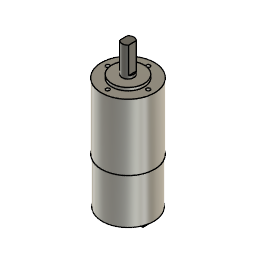
Motor 36GP-3530 (Autodesk Fusion 360 design; units mm, degrees)
Autodesk Fusion 360 part; units mm, degrees
sketch "Sketch1" plane through (0, 0, 0) normal (0, 0, 1) x (1, 0, 0)
  circle A0 centre (0, 0) radius 17.5
  circle A1 centre (0, 0) radius 18
  line L0 (0, 0) -> (11.5, 0) construction
  line L1 (0, 1) -> (0, -1) construction
  line L2 (12, 2) -> (11, 2)
  line L3 (11, 2) -> (11, -2)
  line L4 (11, -2) -> (12, -2)
  line L5 (12, -2) -> (12, 2)
  line L6 (12, 2) -> (11, -2) construction
  line L7 (11, 2) -> (12, -2) construction
  line L8 (-11, 2) -> (-11, -2)
  line L9 (-11, -2) -> (-12, -2)
  line L10 (-12, -2) -> (-12, 2)
  line L11 (-12, 2) -> (-11, 2)
  circle A2 centre (0, 0) radius 11
  circle A3 centre (0, 0) radius 4
  line L12 (-3, 2.6458) -> (-3, -2.6458)
  line L13 (3, -2.6458) -> (3, 2.6458)
  line L14 (3, 2.6458) -> (-3, -2.6458) construction
  line L15 (-3, 2.6458) -> (3, -2.6458) construction
  line L16 (0, 13.7886) -> (-13.7886, 0) construction
  line L17 (-13.7886, 0) -> (0, -13.7886) construction
  line L18 (0, -13.7886) -> (13.7886, 0) construction
  line L19 (13.7886, 0) -> (0, 13.7886) construction
  line L20 (0, 13.7886) -> (0, -13.7886) construction
  line L21 (-13.7886, 0) -> (13.7886, 0) construction
  point P0 (11.5, 0)
  point P1 (-13.7886, 0)
  point P2 (0, 13.7886)
  point P3 (13.7886, 0)
  point P4 (0, -13.7886)
  dimension "d1" = 35
  dimension "d2" = 36
  dimension "d3" = 11.5
  dimension "d4" = 1
  dimension "d5" = 4
  dimension "d6" = 22
  dimension "d7" = 8
  dimension "d8" = 6
  dimension "d9" = 19.5
  dimension "d10" = 19.5
  constraint coincident A0.centre A1.centre
  constraint horizontal L0
  constraint perpendicular L0 L1
  constraint horizontal L2
  constraint perpendicular L2 L3
  constraint parallel L2 L4
  constraint parallel L3 L5
  constraint coincident L6 P0
  constraint coincident L7 P0
  constraint coincident P0 L0.end
  constraint symmetric L1 L2.start L10.end
  constraint symmetric L1 L2.end L8.start
  constraint symmetric L1 L3.end L8.end
  constraint symmetric L1 L4.end L9.end
  constraint concentric A1 A2
  constraint concentric A1 A3
  constraint parallel L12 L13
  constraint coincident L14 A0.centre
  constraint coincident L15 A0.centre
  constraint coincident A3 L13.end
  constraint perpendicular L16 L17
  constraint parallel L16 L18
  constraint parallel L17 L19
  constraint coincident L20 A0.centre
  constraint coincident L21 A0.centre
  constraint coincident P1 L16.end
  constraint coincident P2 L16.start
  constraint coincident P3 L18.end
  constraint coincident P4 L17.end
  measures "d1" diameter of A0
  measures "d2" diameter of A1
  measures "d3" distance of A0.centre P0
  measures "d4" distance of L3.end L4.end
  measures "d5" distance of L2.end L3.end
  measures "d6" diameter of A2
  measures "d7" diameter of A3
  measures "d8" distance of L12.end L13.start
  measures "d9" distance of P4 P3
  measures "d10" distance of P1 P4
extrude "Extrude1" add sketch "Sketch1" against normal blind 45 contours A0 | A1 | L2 L3 L4 L5 | L8 L9 L10 L11 | A2 | A3 L13 | A3 L12 L13 | A3 L12 makes body 1 in component "Gearmotor"
extrude "Extrude2" add sketch "Sketch1" against normal blind 31 from surface at -45 contours A0 | L2 L3 L4 L5 | L8 L9 L10 L11 | A2 | A3 L13 | A3 L12 L13 | A3 L12 bodies 1 in component "Gearmotor"
extrude "Extrude3" add sketch "Sketch1" against normal blind 2.25 from surface at -76 contours A3 L13 | A3 L12 L13 | A3 L12 bodies 1 in component "Gearmotor"
extrude "Extrude4" add sketch "Sketch1" against normal blind 5.3 from surface at -76 contours L2 L3 L4 L5 | L8 L9 L10 L11 bodies 1 in component "Gearmotor"
extrude "Extrude5" add sketch "Sketch1" along normal blind 2 contours A2 bodies 1 in component "Gearmotor"
extrude "Extrude1'" add sketch "Sketch1" along normal blind 22 separate body contours A3 L13 | A3 L12 L13 | A3 L12 makes body 2 in component "Shaft"
extrude "Extrude2'" cut sketch "Sketch1" against normal blind 18 from surface at 22 contours A3 L13 | A3 L12 bodies 2 in component "Shaft"
hole "Hole1" at (-13.7886, 0, 0) at (0, 13.7886, 0) at (13.7886, 0, 0) at (0, -13.7886, 0) direction (0, 0, -1) diameter 2.529 depth 8 tip angle 180 bodies 1 in component "Gearmotor"
thread "Thread1" "ISO Metric profile 3.0 M3x0.5 M3x0.5 6H" thread offset 0 thread depth 7.4 in component "Gearmotor"
component "Gearmotor" placed x (1, 0, 0) y (0, 1, 0) z (0, 0, 1) at (0, 0, 0)
component "Shaft" placed x (1, 0, 0) y (0, 1, 0) z (0, 0, 1) at (0, 0, 0)
